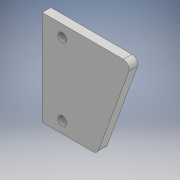
# Autodesk Inventor part: k2_feet
Saved by Autodesk Inventor 2017 (Build 210142000, 142)
## iProperties
Created: 2017-02-15
Part Number: k2_feet
Material: Generic
Document SubType Name: Modeling
Designer: herman
Density: 1 g/cm^3
Appearance: Default
Author: herman
Autodesk Inventor part; units mm, degrees
ref_plane "YZ Plane" through (0, 0, 0) normal (1, 0, 0) x (0, 1, 0)
ref_plane "XZ Plane" through (0, 0, 0) normal (0, 1, 0) x (-1, 0, 0)
ref_plane "XY Plane" through (0, 0, 0) normal (0, 0, 1) x (1, 0, 0)
sketch "Sketch1" plane through (0, 0, 0) normal (0, 1, 0) x (-1, 0, 0)
  line L0 (1.9014, 11.5388) -> (1.9014, -21.4612)
  line L1 (1.9014, -21.4612) -> (-17.0986, -21.4612)
  line L2 (-17.0986, -21.4612) -> (-29.1096, 11.5388)
  line L3 (-29.1096, 11.5388) -> (1.9014, 11.5388)
  line L4 (-17.0986, -21.4612) -> (-17.0986, 11.5388) construction
  point P0 (0, 0)
  dimension "d1" = 33
  dimension "d2" = 20
  dimension "d22" = 19
  constraints: 10 end point, 2 perpendicular, 1 parallel, 1 point on line, 1 vertical
  measures "d1" distance of L0.start L0.end
  measures "d2" angle of L2 L4
  measures "d22" distance of L0.end L1.end
extrude "Extrusion1" add sketch "Sketch1" along normal blind 3
sketch "Sketch3" plane through (0, 0, 0) normal (0, -1, 0) x (1, 0, 0)
  line L0 (29.1096, 11.5388) -> (-1.9014, 11.5388) projected
  line L1 (-1.9014, 11.5388) -> (-1.9014, -21.4612) projected
  line L2 (-1.9014, -21.4612) -> (17.0986, -21.4612) projected
  point P0 (0, 0)
  point P1 (5.0986, 7.5388)
  point P2 (5.0986, -17.4612)
  dimension "d5" = 4
  dimension "d6" = 4
  dimension "d19" = 7
  dimension "d21" = 7
  measures "d5" vertical distance of L0.end point (5.099, 7.539)
  measures "d6" distance from line of L2 point (5.099, -17.461)
  measures "d19" distance from line of L1 point (5.099, -17.461)
  measures "d21" distance from line of L1 point (5.099, 7.539)
hole "Hole1" at (5.0986, 0, 7.5388) at (5.0986, 0, -17.4612) direction (0, 1, 0) diameter 3 end through all
fillet "Fillet1" radius 2 1 edges at (29.1096, 1.5, 11.5388)
fillet "Fillet2" radius 2 1 edges at (17.0986, 1.5, -21.4612)
equation "\"d6\" = d5"
equation "\"d21\" = d19"
body "Solid1"
